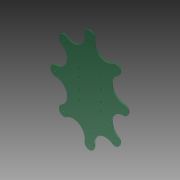
# Autodesk Inventor part: BodyBottom
Saved by Autodesk Inventor 2015 (Build 190159000, 159)
## iProperties
Created: 2015-10-10
Part Number: BodyBottom
Material: Generic
Document SubType Name: Modeling
Designer: styku
Density: 1 g/cm^3
Appearance: Clear - Green 1
Mass: 67.6531 g
Surface Area: 483.612 cm^2
Volume: 67.6531 cm^3
Author: styku
Autodesk Inventor part; units mm, degrees
ref_plane "YZ Plane" through (0, 0, 0) normal (1, 0, 0) x (0, 1, 0)
ref_plane "XZ Plane" through (0, 0, 0) normal (0, 1, 0) x (-1, 0, 0)
ref_plane "XY Plane" through (0, 0, 0) normal (0, 0, 1) x (1, 0, 0)
sketch "Sketch1" plane through (0, 0, 0) normal (0, 1, 0) x (-1, 0, 0)
  line L0 (0, -135) -> (0, 190) construction
  line L1 (111, 0) -> (-155, 0) construction
  ellipse E0 centre (0, 0) end of major axis (0, 110) minor radius 80 construction
  arc A0 (79.5622, -11.4917) -> (91.5, 0) centre (80, 0) ccw
  arc A1 (0, -121.5) -> (11.4442, -108.8687) centre (0, -110) ccw
  arc A2 (53.6974, -81.5386) -> (66.0076, -62.1493) centre (60.3721, -72.1738) ccw
  arc A3 (79.5622, -11.4917) -> (66.0076, -62.1493) centre (79.2711, -38.556) ccw
  arc A4 (53.6974, -81.5386) -> (11.4442, -108.8687) centre (37.9882, -103.5791) ccw
  arc A5 (-91.5, 0) -> (-79.5622, -11.4917) centre (-80, 0) ccw
  arc A6 (-11.4442, -108.8687) -> (0, -121.5) centre (0, -110) ccw
  arc A7 (-66.0076, -62.1493) -> (-53.6974, -81.5386) centre (-60.3721, -72.1738) ccw
  arc A8 (-66.0076, -62.1493) -> (-79.5622, -11.4917) centre (-79.2711, -38.556) ccw
  arc A9 (-11.4442, -108.8687) -> (-53.6974, -81.5386) centre (-37.9882, -103.5791) ccw
  arc A10 (91.5, 0) -> (79.5622, 11.4917) centre (80, 0) ccw
  arc A11 (11.4442, 108.8687) -> (0, 121.5) centre (0, 110) ccw
  arc A12 (66.0076, 62.1493) -> (53.6974, 81.5386) centre (60.3721, 72.1738) ccw
  arc A13 (66.0076, 62.1493) -> (79.5622, 11.4917) centre (79.2711, 38.556) ccw
  arc A14 (11.4442, 108.8687) -> (53.6974, 81.5386) centre (37.9882, 103.5791) ccw
  arc A15 (0, 121.5) -> (-11.4442, 108.8687) centre (0, 110) ccw
  arc A16 (-53.6974, 81.5386) -> (-11.4442, 108.8687) centre (-37.9882, 103.5791) ccw
  arc A17 (-53.6974, 81.5386) -> (-66.0076, 62.1493) centre (-60.3721, 72.1738) ccw
  arc A18 (-79.5622, 11.4917) -> (-66.0076, 62.1493) centre (-79.2711, 38.556) ccw
  arc A19 (-79.5622, 11.4917) -> (-91.5, 0) centre (-80, 0) ccw
  line L2 (53.0109, -83.8154) -> (69.937, -57.0473) construction
  circle A20 centre (56.3638, -78.5129) radius 0.5
  line L3 (66.5644, -76.0894) -> (31.8982, -54.1692) construction
  circle A21 centre (64.3804, -65.8348) radius 0.5
  line L4 (80, -8.2711) -> (80, 9) construction
  circle A22 centre (80, -7.5) radius 0.5
  line L5 (9.0844, -110) -> (-9.2812, -110) construction
  circle A23 centre (7, -110) radius 0.5
  circle A24 centre (-56.3638, -78.5129) radius 0.5
  circle A25 centre (-64.3804, -65.8348) radius 0.5
  circle A26 centre (-80, -7.5) radius 0.5
  circle A27 centre (-7, -110) radius 0.5
  circle A28 centre (56.3638, 78.5129) radius 0.5
  circle A29 centre (64.3804, 65.8348) radius 0.5
  circle A30 centre (80, 7.5) radius 0.5
  circle A31 centre (7, 110) radius 0.5
  circle A32 centre (-7, 110) radius 0.5
  circle A33 centre (-56.3638, 78.5129) radius 0.5
  circle A34 centre (-64.3804, 65.8348) radius 0.5
  circle A35 centre (-80, 7.5) radius 0.5
  circle A36 centre (60.3721, -72.1738) radius 2
  circle A37 centre (0, -110) radius 2
  circle A38 centre (-60.3721, -72.1738) radius 2
  circle A39 centre (80, 0) radius 2
  circle A40 centre (-80, 0) radius 2
  circle A41 centre (60.3721, 72.1738) radius 2
  circle A42 centre (0, 110) radius 2
  circle A43 centre (-60.3721, 72.1738) radius 2
  line L6 (-12.5, 65) -> (-12.5, 74)
  circle A44 centre (50, 0) radius 1.75
  circle A45 centre (35.016, -56.1406) radius 1.75
  circle A46 centre (0, -80) radius 1.75
  circle A47 centre (-50, 0) radius 1.75
  circle A48 centre (-35.016, -56.1406) radius 1.75
  line L7 (66.5644, 76.0894) -> (31.8982, 54.1692) construction
  circle A49 centre (0, 110) radius 2
  circle A50 centre (35.016, 56.1406) radius 1.75
  circle A51 centre (0, 80) radius 1.75
  circle A52 centre (-35.016, 56.1406) radius 1.75
  dimension "d0" = 110
  dimension "d1" = 80
  dimension "d2" = 23
  dimension "d3" = 23
  dimension "d4" = 23
  dimension "d6" = 1
  dimension "d7" = 7.5
  dimension "d8" = 1
  dimension "d9" = 7.5
  dimension "d12" = 1
  dimension "d13" = 7
  dimension "d22" = 4
  dimension "d23" = 4
  dimension "d24" = 4
  dimension "d25" = 4
  dimension "d26" = 4
  dimension "d47" = 3.5
  dimension "d48" = 30
  dimension "d49" = 3.5
  dimension "d50" = 30
  dimension "d51" = 3.5
  dimension "d52" = 30
  constraints: 53 centre point, 49 symmetric about line, 40 point on circle, 16 end point, 15 point on line, 6 coincident, 4 vertical, 3 horizontal, 2 tangent, 1 equal radius, 1 perpendicular, 47 other
  measures "d2" diameter of A0
  measures "d3" diameter of A1
  measures "d4" diameter of A2
  measures "d6" diameter of A20
  measures "d7" distance from line of L3 A20.centre
  measures "d8" diameter of A22
  measures "d9" distance from line of L1 A22.centre
  measures "d12" diameter of A23
  measures "d13" distance from line of L0 A23.centre
  measures "d22" diameter of A36
  measures "d23" diameter of A37
  measures "d24" diameter of A38
  measures "d25" diameter of A39
  measures "d26" diameter of A40
  measures "d47" diameter of A44
  measures "d48" distance of A0.centre A44.centre
  measures "d49" diameter of A45
  measures "d50" distance from line of A45.centre L2
  measures "d51" diameter of A46
  measures "d52" distance of A1.centre A46.centre
extrude "Extrusion7" add sketch "Sketch1" along normal blind 3
sketch "Sketch2" plane through (0, 0, 0) normal (0, -1, 0) x (1, 0, 0)
  line L0 (0, 96) -> (0, -64) construction
  line L1 (-60, 0) -> (61, 0) construction
  line L2 (-26.5, 15) -> (-25, 15)
  line L3 (-25, 15) -> (-25, 10)
  line L4 (-25, 10) -> (-26.5, 10)
  line L5 (-26.5, 10) -> (-26.5, 15)
  line L6 (-26.5, 35) -> (-25, 35)
  line L7 (-25, 35) -> (-25, 30)
  line L8 (-25, 30) -> (-26.5, 30)
  line L9 (-26.5, 30) -> (-26.5, 35)
  line L10 (26.5, 15) -> (25, 15)
  line L11 (25, 15) -> (25, 10)
  line L12 (25, 10) -> (26.5, 10)
  line L13 (26.5, 10) -> (26.5, 15)
  line L14 (26.5, 35) -> (25, 35)
  line L15 (25, 35) -> (25, 30)
  line L16 (25, 30) -> (26.5, 30)
  line L17 (26.5, 30) -> (26.5, 35)
  line L18 (-26.5, -15) -> (-25, -15)
  line L19 (-25, -15) -> (-25, -10)
  line L20 (-25, -10) -> (-26.5, -10)
  line L21 (-26.5, -10) -> (-26.5, -15)
  line L22 (-26.5, -35) -> (-25, -35)
  line L23 (-25, -35) -> (-25, -30)
  line L24 (-25, -30) -> (-26.5, -30)
  line L25 (-26.5, -30) -> (-26.5, -35)
  line L26 (26.5, -15) -> (25, -15)
  line L27 (25, -15) -> (25, -10)
  line L28 (25, -10) -> (26.5, -10)
  line L29 (26.5, -10) -> (26.5, -15)
  line L30 (26.5, -35) -> (25, -35)
  line L31 (25, -35) -> (25, -30)
  line L32 (25, -30) -> (26.5, -30)
  line L33 (26.5, -30) -> (26.5, -35)
  point P0 (0, 0)
  dimension "d57" = 1.5
  dimension "d58" = 5
  dimension "d59" = 25
  dimension "d60" = 10
  dimension "d61" = 1.5
  dimension "d62" = 5
  dimension "d63" = 30
  constraints: 68 end point, 24 symmetric about line, 4 horizontal, 4 parallel, 2 perpendicular, 2 vertical, 1 collinear
  measures "d57" distance of L3.end L4.end
  measures "d58" distance of L2.end L3.end
  measures "d59" distance between parallel lines of L0 L3
  measures "d60" distance between parallel lines of L1 L4
  measures "d61" distance of L7.end L8.end
  measures "d62" distance of L6.end L7.end
  measures "d63" distance between parallel lines of L1 L8
extrude "Extrusion8" cut sketch "Sketch2" against normal blind 31.25
body "Solid4"
